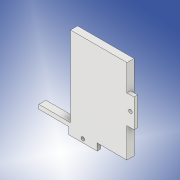
# Autodesk Inventor part: TC005
Saved by Autodesk Inventor 2017 SP1 (Build 210196100, 196)
## iProperties
Created: 2017-08-15
Part Number: TC005
Material: ABS Plastic
Document SubType Name: Modeling
Designer: Zach
Density: 1.06 g/cm^3
Appearance: CR White
Author: Zach
Autodesk Inventor part; units mm, degrees
ref_plane "YZ Plane" through (0, 0, 0) normal (1, 0, 0) x (0, 1, 0)
ref_plane "XZ Plane" through (0, 0, 0) normal (0, 1, 0) x (-1, 0, 0)
ref_plane "XY Plane" through (0, 0, 0) normal (0, 0, 1) x (1, 0, 0)
sketch "Sketch1" plane through (0, 0, 0) normal (0, 0, 1) x (1, 0, 0)
  line L0 (0, 0) -> (124, 0)
  line L1 (124, 0) -> (124, 124)
  line L2 (124, 124) -> (0, 124)
  line L3 (0, 124) -> (0, 0)
  dimension "d0" = 124
  dimension "d1" = 124
  constraints: 8 end point, 2 parallel, 1 horizontal, 1 perpendicular
  measures "d0" distance of L2.end L1.end
  measures "d1" distance of L1.end L0.end
extrude "Extrusion1" add sketch "Sketch1" along normal blind 10
sketch "Sketch2" plane through (0, 0, 10) normal (0, 0, 1) x (1, 0, 0)
  line L0 (124, 0) -> (124, 124) projected
  line L1 (124, 82) -> (134, 82)
  line L2 (134, 82) -> (134, 42)
  line L3 (134, 42) -> (124, 42)
  line L4 (124, 42) -> (124, 82)
  line L5 (0, 0) -> (124, 0) projected
  line L6 (42, 0) -> (82, 0)
  line L7 (82, 0) -> (82, -10)
  line L8 (82, -10) -> (42, -10)
  line L9 (42, -10) -> (42, 0)
  circle A0 centre (129, 62) radius 2.5
  circle A1 centre (62, -5) radius 2.5
  point P0 (129, 82)
  point P1 (62, 0)
  point P2 (62, 0)
  point P3 (62, -10)
  point P4 (134, 62)
  point P5 (124, 62)
  point P6 (124, 62)
  point P7 (42, -5)
  dimension "d4" = 10
  dimension "d5" = 40
  dimension "d6" = 40
  dimension "d7" = 10
  dimension "d8" = 5
  dimension "d9" = 5
  constraints: 16 end point, 8 midpoint, 4 horizontal alignment, 4 parallel, 3 vertical alignment, 2 centre point, 2 horizontal, 2 perpendicular, 2 point on line
  measures "d4" distance of L2.end L3.end
  measures "d5" distance of L1.end L2.end
  measures "d6" distance of L7.end L8.end
  measures "d7" distance of L6.end L7.end
  measures "d8" diameter of A0
  measures "d9" diameter of A1
extrude "Extrusion2" add sketch "Sketch2" against normal blind 5
sketch "Sketch3" plane through (0, 0, 10) normal (0, 0, 1) x (1, 0, 0)
  line L0 (124, 124) -> (0, 124) projected
  line L1 (0, 124) -> (44.5, 124)
  line L2 (44.5, 124) -> (44.5, 6)
  line L3 (44.5, 6) -> (0, 6)
  line L4 (0, 6) -> (0, 124)
  point P0 (0, 0)
  dimension "d12" = 44.5
  dimension "d13" = 118
  constraints: 8 end point, 2 parallel, 1 horizontal, 1 perpendicular
  measures "d12" distance of L2.end L3.end
  measures "d13" distance of L1.end L2.end
extrude "Extrusion3" cut sketch "Sketch3" against normal through all
sketch "Sketch6" plane through (0, 0, 10) normal (0, 0, 1) x (1, 0, 0)
  line L0 (44.5, 124) -> (44.5, 6) projected
  line L1 (124, 0) -> (124, 124) projected
  line L2 (44.5, 124) -> (124, 124)
  line L3 (124, 124) -> (124, 119)
  line L4 (124, 119) -> (44.5, 119)
  line L5 (44.5, 119) -> (44.5, 124)
  point P0 (0, 0)
  dimension "d19" = 5
  constraints: 8 end point, 2 parallel, 1 horizontal, 1 perpendicular, 1 point on line
  measures "d19" distance of L2.end L3.end
extrude "Extrusion5" cut sketch "Sketch6" against normal through all
body "Solid1"
